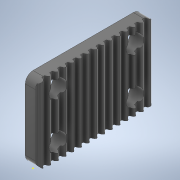
# Autodesk Inventor part: beltpress2
Saved by Autodesk Inventor 2020.2 (Build 242310000, 310)
## iProperties
Created: 2020-08-07
Part Number: beltpress2
Material: Generic
Document SubType Name: Modeling
Designer: JK
Density: 1 g/cm^3
Appearance: Smooth - Black
Author: JK
Autodesk Inventor part; units mm, degrees
ref_plane "YZ Plane" through (0, 0, 0) normal (1, 0, 0) x (0, 1, 0)
ref_plane "XZ Plane" through (0, 0, 0) normal (0, 1, 0) x (-1, 0, 0)
ref_plane "XY Plane" through (0, 0, 0) normal (0, 0, 1) x (1, 0, 0)
sketch "Sketch1" plane through (0, 0, 0) normal (0, 1, 0) x (-1, 0, 0)
  circle A0 centre (0.3248, -1) radius 0.555
  line L0 (1.1618, 2.0652) -> (0.8878, 2.0652)
  line L1 (0.8878, 2.0652) -> (0.8878, -1.6244)
  line L2 (0.8878, -1.6244) -> (1.1618, -1.6244)
  line L3 (1.1618, -1.6244) -> (1.1618, 2.0652)
  circle A1 centre (0.5318, -1.4) radius 1
  line L4 (0.3248, -1) -> (2.1204, -1)
  line L5 (-0.2182, -0.7824) -> (-0.2182, -1.752)
  circle A2 centre (0.3818, -0.2598) radius 0.15
  line L6 (-0.8245, -1) -> (2.3036, -1)
  line L7 (0.5318, -1.4) -> (0.5318, 0.5063)
  line L8 (0.5318, 0) -> (1.1618, 0)
  point P0 (0, 0)
  point P1 (0.5318, -0.2598)
  point P2 (0.4013, -0.4085)
  point P3 (-0.3847, -1)
  point P4 (1.1618, -1)
  dimension "d1" = 1.11
  dimension "d3" = 0.4
  dimension "d4" = 0.75
  dimension "d5" = 1.38
  dimension "d6" = 2
  dimension "d7" = 0.3
  dimension "d9" = 1
  constraints: 18 end point, 4 point on line, 3 centre point, 2 horizontal, 2 parallel, 2 perpendicular, 2 tangent, 2 vertical
  measures "d1" diameter of A0
  measures "d3" distance from line of L4 L7.start
  measures "d4" distance from line of L7.start L5
  measures "d5" distance between parallel lines of L3 L5
  measures "d6" diameter of A1
  measures "d7" diameter of A2
  measures "d9" vertical distance of point (0, 0) L4.start
extrude "Extrusion1" add sketch "Sketch1" along normal blind 20 contours L4 L7 A0 | A0 L7 A1 L1 L4 | L7 L4 L6 L5 A0 A1 | A0 A1 L7 | L1 A1 L3 L4 | L7 L8 L1 A1 | A1 A2 L7 | L6 A1 A0 | A0 L5 L6 | L1 L8 L3 A1 picked at (-0.2204, -0.9361)
mirror "Mirror1" about plane through (0.3847, 0, -1) normal (0, 0, -1) of "Extrusion1"
pattern_linear "Rectangular Pattern1" count 15 spacing 2 along (0, 0, -1) of "Extrusion1", "Mirror1"
sketch "Sketch2" plane through (-1.1618, 0, 0) normal (-1, 0, 0) x (0, 0, 1)
  line L0 (-5, 0) -> (-5, 20) projected
  circle A0 centre (-5, 4) radius 2.25
  circle A1 centre (-25, 4) radius 2.25
  circle A2 centre (-25, 16) radius 2.25
  circle A3 centre (-5, 16) radius 2.25
  line L1 (-30, 0) -> (-30, 20) projected
  line L2 (0, 0) -> (-30, 0) projected
  point P0 (-5, 18.25)
  point P1 (-5, 13.75)
  point P2 (-5, 6.25)
  point P3 (-5, 1.75)
  dimension "d15" = 4.5
  dimension "d16" = 12
  dimension "d17" = 20
  dimension "d18" = 5
  dimension "d19" = 4
  constraints: 4 centre point, 3 equal radius, 2 horizontal alignment, 2 vertical alignment
  measures "d15" diameter of A0
  measures "d16" distance of A0.centre A3.centre
  measures "d17" distance of A1.centre A0.centre
  measures "d18" distance from line of L1 A1.centre
  measures "d19" distance from line of L2 A1.centre
extrude "Extrusion2" cut sketch "Sketch2" against normal blind 10
sketch "Sketch3" plane through (-1.1618, 0, 0) normal (-1, 0, 0) x (0, 0, 1)
  point P0 (0, 0)
sketch "Sketch4" plane through (-1.1618, 0, 0) normal (-1, 0, 0) x (0, 0, 1)
  line L0 (-16.2598, 0) -> (-16.2598, 20) projected
  line L1 (-11.7402, 0) -> (-11.7402, 20) projected
  line L2 (-13.5915, 0) -> (-13.5915, 20) projected
  line L3 (-1.5915, 0) -> (-1.5915, 20) projected
  circle A0 centre (-25, 16) radius 2.25 projected
  circle A1 centre (-25, 4) radius 2.25 projected
  circle A2 centre (-5, 16) radius 2.25 projected
  circle A3 centre (-5, 4) radius 2.25 projected
  line L4 (0, 0) -> (-30, 0) projected
  line L5 (0, 0) -> (0, 20) projected
  line L6 (0, 20) -> (-30, 20) projected
  line L7 (-30, 0) -> (-30, 20) projected
  point P0 (0, 0)
extrude "Extrusion3" add sketch "Sketch4" along normal blind 2
fillet "Fillet1" radius 2 4 edges at (-1.8468, 20, -30) (-1.8468, 20, 0) (-1.8468, 0, 0) (-1.8468, 0, -30)
body "Solid1"
